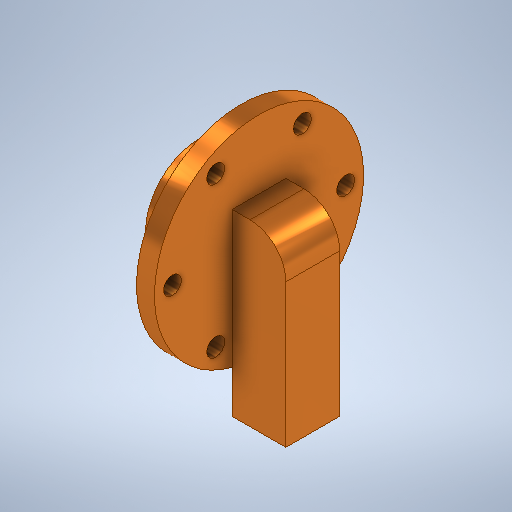
# Autodesk Inventor part: 155 part 1
Saved by Autodesk Inventor 2025.1 (Build 291241000, 241)
## iProperties
Created: 2024-08-03
Part Number: 155 part 1
Material: Gold
Document SubType Name: Modeling
Designer: ffogue
Density: 19.3 g/cm^3
Appearance: Metal 1600F Hot
Author: ffogue
Autodesk Inventor part; units mm, degrees
note: some values were not read from the file. Chosen so that the rebuilt part matches the saved one: direction of "Hole3".
ref_plane "YZ Plane" through (0, 0, 0) normal (1, 0, 0) x (0, 1, 0)
ref_plane "XZ Plane" through (0, 0, 0) normal (0, 1, 0) x (-1, 0, 0)
sketch "Sketch1" plane through (0, 0, 0) normal (0, 0, 1) x (1, 0, 0)
  line L0 (0, 0) -> (0, 9)
  line L1 (0, 9) -> (7, 9)
  line L2 (7, 9) -> (7, 17.5)
  line L3 (7, 17.5) -> (10, 17.5)
  line L4 (10, 17.5) -> (10, 0)
  line L5 (10, 0) -> (0, 0)
  dimension "d0" = 18
  dimension "d1" = 35
  dimension "d2" = 7
  dimension "d3" = 3
  constraints: 12 end point, 5 perpendicular, 1 vertical
  measures "d0" diameter of L1 L5
  measures "d1" diameter of L3.end L5
  measures "d2" distance of L0.end L1.end
  measures "d3" distance of L2.end L3.end
revolve "Revolution1" add sketch "Sketch1" angle 360 about axis through (10, 0, 0) along (-1, 0, 0)
sketch "Sketch2" plane through (0, 0, 0) normal (0, 1, 0) x (-1, 0, 0)
  line L0 (-10, -17.5) -> (-10, 17.5) projected
  line L1 (-10, 6) -> (-13, 6)
  line L2 (-19, 0) -> (-19, -24)
  line L3 (-19, -24) -> (-10, -24)
  line L4 (-10, -24) -> (-10, 6)
  line L5 (-10, -17.5) -> (-7, -17.5) projected
  arc A0 (-13, 6) -> (-19, 0) centre (-13, 0) ccw
  point P0 (0, 0)
  point P1 (-8.5, -17.5)
  dimension "d6" = 30
  dimension "d7" = 9
  dimension "d8" = 6.5
  dimension "d9" = 6
  constraints: 8 end point, 2 parallel, 2 point on circle, 2 tangent, 1 centre point, 1 horizontal, 1 midpoint, 1 perpendicular, 1 point on line
  measures "d6" distance between parallel lines of L1 L3
  measures "d7" distance of L2.end L3.end
  measures "d8" distance from line of point (-8.5, -17.5) L3
  measures "d9" radius of A0
extrude "Extrusion1" add sketch "Sketch2" along normal mid plane 9
sketch "Sketch3" plane through (19, 4.5, -24) normal (0, 0, -1) x (-1, 0, 0)
  line L0 (9, 0) -> (9, -9) projected
  line L1 (0, 0) -> (9, 0) projected
  point P0 (19, -4.5)
  point P1 (4.5, -4.5)
  point P2 (9, -4.5)
  dimension "d19" = 4.5
  dimension "d20" = 4.5
  constraints: 1 midpoint
  measures "d19" distance of point (9, -4.5) point (4.5, -4.5)
  measures "d20" distance from line of L1 point (4.5, -4.5)
hole "Hole1" at (14.5, 0, -24) direction (0, 0, 1) diameter 4.917 depth 18 counterbore diameter 6 counterbore depth 7 thread size "M6x1" class "6H" standard "ISO Metric profile"
ref_plane "Work Plane1" through (0, 0, -7.5) normal (0, 0, 1) x (1, 0, 0)
sketch "Sketch4" plane through (0, 0, -7.5) normal (0, 0, 1) x (1, 0, 0)
  circle A0 centre (14.5, 0) radius 3 projected
  point P0 (0, 0)
  constraints: 1 coincident
hole "Hole2" at (14.5, 0, -7.5) direction (0, 0, 1) diameter 1.5 depth 7.5
sketch "Sketch5" plane through (10, 0, 0) normal (1, 0, 0) x (0, 0, -1)
  line L0 (-6, 4.5) -> (16.9115, 4.5) projected
  arc A0 (16.9115, 4.5) -> (16.9115, -4.5) centre (0, 0) ccw projected
  line L1 (16.9115, -4.5) -> (-6, -4.5) projected
  line L2 (-6, -4.5) -> (-6, 4.5) projected
  circle A1 centre (0, 0) radius 14.5 construction
  line L3 (0, -4.5) -> (0, 4.5) projected
  line L4 (0, 0) -> (12.5574, 7.25) construction
  line L5 (0, 0) -> (27.6817, 0) construction
  dimension "d29" = 29
  dimension "d30" = 30
  constraints: 4 end point, 2 coincident, 2 midpoint, 1 horizontal, 3 other
  measures "d30" angle of L5 L4
hole "Hole3" at (10, 7.25, -12.5574) direction (-1, 0, 0) diameter 3 depth 3
pattern_circular "Circular Pattern1" count 6 over 360 about axis through (8.5, 0, 0) along (-1, 0, 0) of "Hole3"
sketch "Sketch6" plane through (0, 0, 0) normal (-1, 0, 0) x (0, 0, 1)
  circle A0 centre (0, 0) radius 9 projected
  constraints: 1 coincident
hole "Hole4" at (0, 0, 0) direction (1, 0, 0) diameter 1.5 depth 14.5
body "Solid1"
